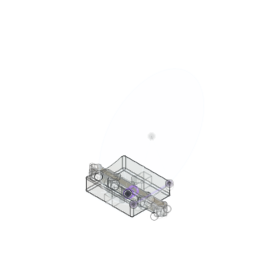
AdjustableDumbbellStand (Autodesk Fusion 360 design; units mm, degrees)
Autodesk Fusion 360 part; units mm, degrees
sketch "Sketch1" plane through (0, 0, 0) normal (0, 0, 1) x (1, 0, 0) in component "Connector"
  line L0 (124.9, -14.9) -> (-124.9, -14.9)
  line L1 (-124.9, -14.9) -> (-124.9, 14.9)
  line L2 (-124.9, 14.9) -> (124.9, 14.9)
  line L3 (124.9, 14.9) -> (124.9, -14.9)
  line L4 (124.9, -14.9) -> (-124.9, 14.9) construction
  line L5 (-124.9, -14.9) -> (124.9, 14.9) construction
  line L6 (124.9, 24.9) -> (124.9, -24.9)
  line L7 (0, 0) -> (144.7, 0) construction
  line L8 (124.9, 24.9) -> (144.7, 0)
  line L9 (124.9, -24.9) -> (144.7, 0)
  line L10 (0, 2.5) -> (0, 20)
  line L11 (-124.9, 24.9) -> (-144.7, 0)
  line L12 (-124.9, -24.9) -> (-144.7, 0)
  line L13 (-124.9, 24.9) -> (-124.9, -24.9)
  line L14 (-124.9, -24.9) -> (-105.1, 0)
  line L15 (-124.9, 24.9) -> (-105.1, 0)
  line L16 (124.9, 24.9) -> (105.1, 0)
  line L17 (124.9, -24.9) -> (105.1, 0)
  dimension "d1" = 249.8
  dimension "d2" = 29.8
  dimension "d3" = 49.8
  dimension "d24" = 19.8
  constraint horizontal L0
  constraint perpendicular L0 L1
  constraint parallel L0 L2
  constraint parallel L1 L3
  constraint coincident L4 L7.start
  constraint coincident L5 L7.start
  constraint coincident L7.start origin
  constraint parallel L3 L6
  constraint collinear L3 L6
  constraint equal L8 L9
  constraint horizontal L7
  constraint symmetric L6.start L10 L11.start
  constraint symmetric L6.end L10 L12.start
  constraint symmetric L7.end L10 L11.end
  constraint symmetric L11.start L13 L15.start
  constraint symmetric L11.end L13 L14.end
  constraint symmetric L12.start L13 L14.start
  constraint symmetric L3 L6.start L8.start
  constraint symmetric L3 L6.end L9.start
  constraint symmetric L3 L7.end L16.end
  constraint collinear L1 L13
  measures "d1" distance of L1.end L2.end
  measures "d2" distance of L0.end L1.end
  measures "d3" distance of L6.start L6.end
  measures "d24" distance of L6 L7.end
extrude "Extrude1" add sketch "Sketch1" along normal blind 28.8 makes body 1 in component "Connector"
fillet "Fillet1" radius 6 10 edges at (-144.7, 0, 14.4) (144.7, 0, 14.4) (116.9482, 14.9, 14.4) (124.9, 24.9, 14.4) (-116.9482, 14.9, 14.4) (-124.9, 24.9, 14.4) (124.9, -24.9, 14.4) (116.9482, -14.9, 14.4) (-124.9, -24.9, 14.4) (-116.9482, -14.9, 14.4) on bodies 1 in component "Connector"
chamfer "Chamfer1" distance 5 angle 45 1 faces at (-38.0179, -4.9667, 28.8) on bodies 1 in component "Connector"
sketch "Sketch1 (2)" plane through (0, 0, 0) normal (0, 0, 1) x (1, 0, 0) in component "Base"
  line L0 (-90, 75) -> (90, 75)
  line L1 (90, 75) -> (90, -75)
  line L2 (90, -75) -> (-90, -75)
  line L3 (-90, -75) -> (-90, 75)
  line L4 (-90, 75) -> (90, -75) construction
  line L5 (90, 75) -> (-90, -75) construction
  line L6 (0, 0) -> (-90, 0) construction
  line L7 (0, 0) -> (0, -75) construction
  dimension "d10" = 180
  dimension "d11" = 150
  constraint horizontal L0
  constraint perpendicular L0 L1
  constraint parallel L0 L2
  constraint parallel L1 L3
  constraint coincident L4 L6.start
  constraint coincident L5 L6.start
  constraint coincident L6.start L7.start
  constraint midpoint L3 L6.end
  constraint midpoint L2 L7.end
  measures "d10" distance of L1.end L2.end
  measures "d11" distance of L0.end L1.end
extrude "Extrude1'" add sketch "Sketch1 (2)" along normal blind 50 separate body makes body 2 in component "Base"
fillet "Fillet1'" radius 6 4 edges at (90, 75, 25) (-90, 75, 25) (-90, -75, 25) (90, -75, 25) on bodies 2 in component "Base"
chamfer "Chamfer1'" distance 5 angle 45 2 faces at (28, -25, 0) (28, -25, 50) on bodies 2 in component "Base"
sketch "Sketch2" plane through (90, 0, 0) normal (1, 0, 0) x (0, 1, 0) in component "Base"
  line L0 (69, 45) -> (-69, 45)
  line L1 (-69, 45) -> (-69, 5)
  line L2 (-69, 5) -> (69, 5)
  line L3 (69, 5) -> (69, 45)
  line L4 (-69, 45) -> (69, 45)
  line L5 (-69, 45) -> (0, 235) construction
  line L6 (0, 235) -> (69, 45) construction
  circle A0 centre (0, 235) radius 200
  line L7 (-69, 35) -> (69, 35) construction
  line L8 (-69, 45) -> (-69, 35) construction
  dimension "d17" = 400
  dimension "d18" = 10
  constraint coincident L0.end L1.start
  constraint coincident L0.start L3.end
  constraint equal L5 L6
  constraint coincident L5.end L6.start
  constraint perpendicular L1 L7
  constraint equal L0 L7
  constraint perpendicular L0 L8
  constraint tangent A0 L7
  measures "d17" diameter of A0
  measures "d18" distance of L0.end L7.start
extrude "Extrude2" cut sketch "Sketch2" against normal through all contours L0 L4 A0 | L0 L4 A0 bodies 2 in component "Base"
sketch "Sketch1 (3)" plane through (0, 0, 0) normal (0, 0, 1) x (1, 0, 0) in component "ConnectorTip"
  line L0 (0, 0) -> (0, -24.9) construction
  line L1 (0, 0) -> (0, 24.9) construction
  line L2 (0, 0) -> (19.8, 0) construction
  line L3 (0, 0) -> (-19.8, 0) construction
  line L4 (0, -24.9) -> (19.8, 0)
  line L5 (0, 24.9) -> (19.8, 0)
  line L6 (0, 24.9) -> (-19.8, 0)
  line L7 (0, -24.9) -> (-19.8, 0)
  line L8 (-7.9518, -14.9) -> (-37.7518, -14.9)
  line L9 (-37.7518, -14.9) -> (-37.7518, 14.9)
  line L10 (-37.7518, 14.9) -> (-7.9518, 14.9)
  line L11 (-7.9518, 14.9) -> (-7.9518, -14.9)
  dimension "d33" = 24.9
  dimension "d34" = 19.8
  dimension "d39" = 29.8
  constraint coincident L0.start L1.start
  constraint vertical L0
  constraint parallel L0 L1
  constraint equal L0 L1
  constraint perpendicular L1 L2
  constraint perpendicular L1 L3
  constraint equal L2 L3
  constraint horizontal L8
  constraint vertical L9
  constraint horizontal L10
  constraint vertical L11
  constraint coincident L7 L8.start
  constraint coincident L6 L10.end
  constraint equal L8 L11
  measures "d33" distance of L0.start L0.end
  measures "d34" distance of L0.start L2.end
  measures "d39" distance of L8.start L10.end
extrude "Extrude1''" add sketch "Sketch1 (3)" along normal blind 28.8 separate body makes body 3 in component "ConnectorTip"
fillet "Fillet1''" radius 6 3 edges at (0, 24.9, 14.4) (19.8, 0, 14.4) (0, -24.9, 14.4) on bodies 3 in component "ConnectorTip"
sketch "Sketch1 (4)" plane through (0, 0, 0) normal (0, 0, 1) x (1, 0, 0) in component "Base (1)"
  line L0 (-90, 75) -> (90, 75)
  line L1 (90, 75) -> (90, -75)
  line L2 (90, -75) -> (-90, -75)
  line L3 (-90, -75) -> (-90, 75)
  line L4 (-90, 75) -> (90, -75) construction
  line L5 (90, 75) -> (-90, -75) construction
  line L6 (0, 0) -> (-90, 0) construction
  line L7 (0, 0) -> (0, -75) construction
  dimension "d10_1" = 180
  dimension "d11_1" = 150
  constraint horizontal L0
  constraint perpendicular L0 L1
  constraint parallel L0 L2
  constraint parallel L1 L3
  constraint coincident L4 L6.start
  constraint coincident L5 L6.start
  constraint coincident L6.start L7.start
  constraint midpoint L3 L6.end
  constraint midpoint L2 L7.end
  measures "d10_1" distance of L1.end L2.end
  measures "d11_1" distance of L0.end L1.end
extrude "Extrude1'''" add sketch "Sketch1 (4)" along normal blind 50 separate body makes body 4 in component "Base (1)"
fillet "Fillet1'''" radius 6 4 edges at (90, 75, 25) (-90, 75, 25) (-90, -75, 25) (90, -75, 25) on bodies 4 in component "Base (1)"
chamfer "Chamfer1''" distance 5 angle 45 2 faces at (28, -25, 0) (28, -25, 50) on bodies 4 in component "Base (1)"
sketch "Sketch2 (2)" plane through (90, 0, 0) normal (1, 0, 0) x (0, 1, 0) in component "Base (1)"
  line L0 (69, 45) -> (-69, 45)
  line L1 (-69, 45) -> (-69, 5)
  line L2 (-69, 5) -> (69, 5)
  line L3 (69, 5) -> (69, 45)
  line L4 (-69, 45) -> (69, 45)
  line L5 (-69, 45) -> (0, 235) construction
  line L6 (0, 235) -> (69, 45) construction
  circle A0 centre (0, 235) radius 200
  line L7 (-69, 35) -> (69, 35) construction
  line L8 (-69, 45) -> (-69, 35) construction
  dimension "d17_1" = 400
  dimension "d18_1" = 10
  constraint coincident L0.end L1.start
  constraint coincident L0.start L3.end
  constraint equal L5 L6
  constraint coincident L5.end L6.start
  constraint perpendicular L1 L7
  constraint equal L0 L7
  constraint perpendicular L0 L8
  constraint tangent A0 L7
  measures "d17_1" diameter of A0
  measures "d18_1" distance of L0.end L7.start
extrude "Extrude2'" cut sketch "Sketch2 (2)" against normal through all contours L0 L4 A0 | L0 L4 A0 bodies 4 in component "Base (1)"
sketch "Sketch1 (5)" plane through (0, 0, 0) normal (0, 0, 1) x (1, 0, 0) in component "ConnectorTip (1)"
  line L0 (0, 0) -> (0, -24.9) construction
  line L1 (0, 0) -> (0, 24.9) construction
  line L2 (0, 0) -> (19.8, 0) construction
  line L3 (0, 0) -> (-19.8, 0) construction
  line L4 (0, -24.9) -> (19.8, 0)
  line L5 (0, 24.9) -> (19.8, 0)
  line L6 (0, 24.9) -> (-19.8, 0)
  line L7 (0, -24.9) -> (-19.8, 0)
  line L8 (-7.9518, -14.9) -> (-37.7518, -14.9)
  line L9 (-37.7518, -14.9) -> (-37.7518, 14.9)
  line L10 (-37.7518, 14.9) -> (-7.9518, 14.9)
  line L11 (-7.9518, 14.9) -> (-7.9518, -14.9)
  dimension "d33_1" = 24.9
  dimension "d34_1" = 19.8
  dimension "d39_1" = 29.8
  constraint coincident L0.start L1.start
  constraint vertical L0
  constraint parallel L0 L1
  constraint equal L0 L1
  constraint perpendicular L1 L2
  constraint perpendicular L1 L3
  constraint equal L2 L3
  constraint horizontal L8
  constraint vertical L9
  constraint horizontal L10
  constraint vertical L11
  constraint coincident L7 L8.start
  constraint coincident L6 L10.end
  constraint equal L8 L11
  measures "d33_1" distance of L0.start L0.end
  measures "d34_1" distance of L0.start L2.end
  measures "d39_1" distance of L8.start L10.end
extrude "Extrude1''''" add sketch "Sketch1 (5)" along normal blind 28.8 separate body makes body 5 in component "ConnectorTip (1)"
fillet "Fillet1''''" radius 6 3 edges at (0, 24.9, 14.4) (19.8, 0, 14.4) (0, -24.9, 14.4) on bodies 5 in component "ConnectorTip (1)"
sketch "Sketch1 (6)" plane through (0, 0, 0) normal (0, 0, 1) x (1, 0, 0) in component "ConnectorTip (2)"
  line L0 (0, 0) -> (0, -24.9) construction
  line L1 (0, 0) -> (0, 24.9) construction
  line L2 (0, 0) -> (19.8, 0) construction
  line L3 (0, 0) -> (-19.8, 0) construction
  line L4 (0, -24.9) -> (19.8, 0)
  line L5 (0, 24.9) -> (19.8, 0)
  line L6 (0, 24.9) -> (-19.8, 0)
  line L7 (0, -24.9) -> (-19.8, 0)
  line L8 (-7.9518, -14.9) -> (-37.7518, -14.9)
  line L9 (-37.7518, -14.9) -> (-37.7518, 14.9)
  line L10 (-37.7518, 14.9) -> (-7.9518, 14.9)
  line L11 (-7.9518, 14.9) -> (-7.9518, -14.9)
  dimension "d33_2" = 24.9
  dimension "d34_2" = 19.8
  dimension "d39_2" = 29.8
  constraint coincident L0.start L1.start
  constraint vertical L0
  constraint parallel L0 L1
  constraint equal L0 L1
  constraint perpendicular L1 L2
  constraint perpendicular L1 L3
  constraint equal L2 L3
  constraint horizontal L8
  constraint vertical L9
  constraint horizontal L10
  constraint vertical L11
  constraint coincident L7 L8.start
  constraint coincident L6 L10.end
  constraint equal L8 L11
  measures "d33_2" distance of L0.start L0.end
  measures "d34_2" distance of L0.start L2.end
  measures "d39_2" distance of L8.start L10.end
extrude "Extrude1'''''" add sketch "Sketch1 (6)" along normal blind 28.8 separate body makes body 6 in component "ConnectorTip (2)"
fillet "Fillet1'''''" radius 6 3 edges at (0, 24.9, 14.4) (19.8, 0, 14.4) (0, -24.9, 14.4) on bodies 6 in component "ConnectorTip (2)"
combine "Combine10" operation cut target body 4 tool bodies 6 5 body 6 seen with x (1, 0, 0) y (0, 1, 0) z (0, 0, 1) at (-52.2482, 0, 0) body 5 seen with x (0, -1, 0) y (1, 0, 0) z (0, 0, 1) at (0, 37.2482, 0) in component "Base (1)"
sketch "Sketch1 (7)" plane through (0, 0, 0) normal (0, 0, 1) x (1, 0, 0) in component "Base (2)"
  line L0 (-90, 75) -> (90, 75)
  line L1 (90, 75) -> (90, -75)
  line L2 (90, -75) -> (-90, -75)
  line L3 (-90, -75) -> (-90, 75)
  line L4 (-90, 75) -> (90, -75) construction
  line L5 (90, 75) -> (-90, -75) construction
  line L6 (0, 0) -> (-90, 0) construction
  line L7 (0, 0) -> (0, -75) construction
  dimension "d10_2" = 180
  dimension "d11_2" = 150
  constraint horizontal L0
  constraint perpendicular L0 L1
  constraint parallel L0 L2
  constraint parallel L1 L3
  constraint coincident L4 L6.start
  constraint coincident L5 L6.start
  constraint coincident L6.start L7.start
  constraint midpoint L3 L6.end
  constraint midpoint L2 L7.end
  measures "d10_2" distance of L1.end L2.end
  measures "d11_2" distance of L0.end L1.end
extrude "Extrude1''''''" add sketch "Sketch1 (7)" along normal blind 50 separate body makes body 7 in component "Base (2)"
fillet "Fillet1''''''" radius 6 4 edges at (90, 75, 25) (-90, 75, 25) (-90, -75, 25) (90, -75, 25) on bodies 7 in component "Base (2)"
chamfer "Chamfer1'''" distance 5 angle 45 2 faces at (28, -25, 0) (28, -25, 50) on bodies 7 in component "Base (2)"
sketch "Sketch2 (3)" plane through (90, 0, 0) normal (1, 0, 0) x (0, 1, 0) in component "Base (2)"
  line L0 (69, 45) -> (-69, 45)
  line L1 (-69, 45) -> (-69, 5)
  line L2 (-69, 5) -> (69, 5)
  line L3 (69, 5) -> (69, 45)
  line L4 (-69, 45) -> (69, 45)
  line L5 (-69, 45) -> (0, 235) construction
  line L6 (0, 235) -> (69, 45) construction
  circle A0 centre (0, 235) radius 200
  line L7 (-69, 35) -> (69, 35) construction
  line L8 (-69, 45) -> (-69, 35) construction
  dimension "d17_2" = 400
  dimension "d18_2" = 10
  constraint coincident L0.end L1.start
  constraint coincident L0.start L3.end
  constraint equal L5 L6
  constraint coincident L5.end L6.start
  constraint perpendicular L1 L7
  constraint equal L0 L7
  constraint perpendicular L0 L8
  constraint tangent A0 L7
  measures "d17_2" diameter of A0
  measures "d18_2" distance of L0.end L7.start
extrude "Extrude2''" cut sketch "Sketch2 (3)" against normal through all contours L0 L4 A0 | L0 L4 A0 bodies 7 in component "Base (2)"
sketch "Sketch1 (8)" plane through (0, 0, 0) normal (0, 0, 1) x (1, 0, 0) in component "ConnectorTip (3)"
  line L0 (0, 0) -> (0, -24.9) construction
  line L1 (0, 0) -> (0, 24.9) construction
  line L2 (0, 0) -> (19.8, 0) construction
  line L3 (0, 0) -> (-19.8, 0) construction
  line L4 (0, -24.9) -> (19.8, 0)
  line L5 (0, 24.9) -> (19.8, 0)
  line L6 (0, 24.9) -> (-19.8, 0)
  line L7 (0, -24.9) -> (-19.8, 0)
  line L8 (-7.9518, -14.9) -> (-37.7518, -14.9)
  line L9 (-37.7518, -14.9) -> (-37.7518, 14.9)
  line L10 (-37.7518, 14.9) -> (-7.9518, 14.9)
  line L11 (-7.9518, 14.9) -> (-7.9518, -14.9)
  dimension "d33_3" = 24.9
  dimension "d34_3" = 19.8
  dimension "d39_3" = 29.8
  constraint coincident L0.start L1.start
  constraint vertical L0
  constraint parallel L0 L1
  constraint equal L0 L1
  constraint perpendicular L1 L2
  constraint perpendicular L1 L3
  constraint equal L2 L3
  constraint horizontal L8
  constraint vertical L9
  constraint horizontal L10
  constraint vertical L11
  constraint coincident L7 L8.start
  constraint coincident L6 L10.end
  constraint equal L8 L11
  measures "d33_3" distance of L0.start L0.end
  measures "d34_3" distance of L0.start L2.end
  measures "d39_3" distance of L8.start L10.end
extrude "Extrude1'''''''" add sketch "Sketch1 (8)" along normal blind 28.8 separate body makes body 8 in component "ConnectorTip (3)"
fillet "Fillet1'''''''" radius 6 3 edges at (0, 24.9, 14.4) (19.8, 0, 14.4) (0, -24.9, 14.4) on bodies 8 in component "ConnectorTip (3)"
sketch "Sketch1 (9)" plane through (0, 0, 0) normal (0, 0, 1) x (1, 0, 0) in component "ConnectorTip (4)"
  line L0 (0, 0) -> (0, -24.9) construction
  line L1 (0, 0) -> (0, 24.9) construction
  line L2 (0, 0) -> (19.8, 0) construction
  line L3 (0, 0) -> (-19.8, 0) construction
  line L4 (0, -24.9) -> (19.8, 0)
  line L5 (0, 24.9) -> (19.8, 0)
  line L6 (0, 24.9) -> (-19.8, 0)
  line L7 (0, -24.9) -> (-19.8, 0)
  line L8 (-7.9518, -14.9) -> (-37.7518, -14.9)
  line L9 (-37.7518, -14.9) -> (-37.7518, 14.9)
  line L10 (-37.7518, 14.9) -> (-7.9518, 14.9)
  line L11 (-7.9518, 14.9) -> (-7.9518, -14.9)
  dimension "d33_4" = 24.9
  dimension "d34_4" = 19.8
  dimension "d39_4" = 29.8
  constraint coincident L0.start L1.start
  constraint vertical L0
  constraint parallel L0 L1
  constraint equal L0 L1
  constraint perpendicular L1 L2
  constraint perpendicular L1 L3
  constraint equal L2 L3
  constraint horizontal L8
  constraint vertical L9
  constraint horizontal L10
  constraint vertical L11
  constraint coincident L7 L8.start
  constraint coincident L6 L10.end
  constraint equal L8 L11
  measures "d33_4" distance of L0.start L0.end
  measures "d34_4" distance of L0.start L2.end
  measures "d39_4" distance of L8.start L10.end
extrude "Extrude1''''''''" add sketch "Sketch1 (9)" along normal blind 28.8 separate body makes body 9 in component "ConnectorTip (4)"
fillet "Fillet1''''''''" radius 6 3 edges at (0, 24.9, 14.4) (19.8, 0, 14.4) (0, -24.9, 14.4) on bodies 9 in component "ConnectorTip (4)"
combine "Combine10'" operation cut target body 7 tool bodies 9 8 body 9 seen with x (1, 0, 0) y (0, 1, 0) z (0, 0, 1) at (-52.2482, 0, 0) body 8 seen with x (0, 1, 0) y (-1, 0, 0) z (0, 0, 1) at (0, -37.2482, 0) in component "Base (2)"
sketch "Sketch1 (10)" plane through (0, 0, 0) normal (0, 0, 1) x (1, 0, 0) in component "Connector_Extender_A_Full_Length"
  line L0 (124.9, -14.9) -> (-124.9, -14.9)
  line L1 (-124.9, -14.9) -> (-124.9, 14.9) construction
  line L2 (-124.9, 14.9) -> (124.9, 14.9)
  line L3 (124.9, 14.9) -> (124.9, -14.9)
  line L4 (124.9, -14.9) -> (-124.9, 14.9) construction
  line L5 (-124.9, -14.9) -> (124.9, 14.9) construction
  line L6 (124.9, 24.9) -> (124.9, -24.9)
  line L7 (0, 0) -> (144.7, 0) construction
  line L8 (124.9, 24.9) -> (144.7, 0)
  line L9 (124.9, -24.9) -> (144.7, 0)
  line L10 (0, 2.5) -> (0, 20)
  line L11 (124.9, -24.9) -> (105.1, 0)
  line L12 (124.9, 24.9) -> (105.1, 0)
  circle A0 centre (-119.9333, -9.9333) radius 4.9667
  circle A1 centre (-119.9333, 9.9333) radius 4.9667
  circle A2 centre (-112.4833, 0) radius 7.45 construction
  arc A3 (-116.9534, -5.96) -> (-116.9534, 5.96) centre (-112.4835, 0) ccw
  line L13 (-124.9, -14.9) -> (-124.9, -9.9333)
  line L14 (-124.9, 9.9333) -> (-124.9, 14.9)
  circle A4 centre (-129.8667, -9.9333) radius 4.9667
  circle A5 centre (-129.8667, 9.9333) radius 4.9667
  circle A6 centre (-137.3167, 0) radius 7.45
  dimension "d1_1" = 249.8
  dimension "d2_1" = 29.8
  dimension "d3_1" = 49.8
  dimension "d24_1" = 19.8
  dimension "d56" = 9.9333
  dimension "d57" = 14.9
  constraint horizontal L0
  constraint perpendicular L0 L1
  constraint parallel L0 L2
  constraint parallel L1 L3
  constraint coincident L4 L7.start
  constraint coincident L5 L7.start
  constraint coincident L7.start origin
  constraint parallel L3 L6
  constraint equal L8 L9
  constraint horizontal L7
  constraint symmetric L3 L6.start L8.start
  constraint symmetric L3 L6.end L9.start
  constraint symmetric L3 L7.end L11.end
  constraint tangent L0 A0
  constraint tangent L1 A0
  constraint symmetric L7 A0 A1
  constraint tangent A0 A2
  constraint tangent A1 A2
  constraint tangent A1 A3
  constraint coincident A1 A3.end
  constraint coincident A2 A3.end
  constraint coincident A0 A3.start
  constraint coincident A2 A3.start
  constraint coincident L1 L13.end
  constraint coincident A0 L13.end
  constraint coincident A1 L14.start
  constraint coincident L1 L14.start
  constraint symmetric L1 A0 A4
  constraint symmetric L1 A1 A5
  constraint symmetric L1 A2 A6
  constraint coincident L6 L9.start
  measures "d1_1" distance of L1.end L2.end
  measures "d2_1" distance of L0.end L1.end
  measures "d3_1" distance of L6.start L6.end
  measures "d24_1" distance of L6 L7.end
  measures "d56" diameter of A0
  measures "d57" diameter of A2
extrude "Extrude1'''''''''" add sketch "Sketch1 (10)" along normal blind 28.8 separate body contours L0 L6 L11 | L0 L2 L3 L6 L11 L12 | L3 L6 L8 L9 | L0 L2 L11 L12 A0 A1 A3 | L2 L6 L12 | L0 A0 L13 | A0 | A0 A1 A3 A4 A5 A6 | A6 | L2 A1 L14 | A1 makes body 10 in component "Connector_Extender_A_Full_Length"
fillet "Fillet1'''''''''" radius 6 5 edges at (144.7, 0, 14.4) (124.9, 24.9, 14.4) (116.9482, 14.9, 14.4) (124.9, -24.9, 14.4) (116.9482, -14.9, 14.4) on bodies 10 in component "Connector_Extender_A_Full_Length"
chamfer "Chamfer1''''" distance 5 angle 45 7 edges at (-3.9759, 14.9, 28.8) (-3.9759, -14.9, 28.8) (135.6634, -11.3642, 28.8) (143.0343, 0, 28.8) (135.6634, 11.3642, 28.8) (119.4768, -18.0799, 28.8) (119.4768, 18.0799, 28.8) on bodies 10 in component "Connector_Extender_A_Full_Length"
sketch "Sketch1 (11)" plane through (0, 0, 0) normal (0, 0, 1) x (1, 0, 0) in component "Connector_Extender_C_Full_Length"
  line L0 (124.9, -14.9) -> (-124.9, -14.9)
  line L1 (-124.9, -14.9) -> (-124.9, 14.9) construction
  line L2 (-124.9, 14.9) -> (124.9, 14.9)
  line L3 (124.9, 14.9) -> (124.9, -14.9)
  line L4 (124.9, -14.9) -> (-124.9, 14.9) construction
  line L5 (-124.9, -14.9) -> (124.9, 14.9) construction
  line L6 (0, 0) -> (124.9, 0) construction
  line L7 (0, 2.5) -> (0, 20)
  circle A0 centre (-119.9333, -9.9333) radius 4.9667
  circle A1 centre (-119.9333, 9.9333) radius 4.9667
  circle A2 centre (-112.4833, 0) radius 7.45 construction
  arc A3 (-116.9533, -5.96) -> (-116.9533, 5.96) centre (-112.4833, 0) ccw
  line L8 (-124.9, -14.9) -> (-124.9, -9.9333)
  line L9 (-124.9, 9.9333) -> (-124.9, 14.9)
  arc A4 (116.9533, 5.96) -> (116.9533, -5.96) centre (112.4833, 0) ccw construction
  circle A5 centre (119.9333, -9.9333) radius 4.9667 construction
  circle A6 centre (119.9333, 9.9333) radius 4.9667 construction
  circle A7 centre (129.8667, -9.9333) radius 4.9667 construction
  circle A8 centre (129.8667, 9.9333) radius 4.9667 construction
  arc A9 (132.8467, -5.96) -> (132.8467, 5.96) centre (137.3167, 0) ccw
  arc A10 (132.8467, -5.96) -> (124.9, -9.9333) centre (129.8667, -9.9333) ccw
  arc A11 (124.9, 9.9333) -> (132.8467, 5.96) centre (129.8667, 9.9333) ccw
  point P0 (-124.9, 0)
  dimension "d1_1_1" = 249.8
  dimension "d2_1_1" = 29.8
  dimension "d56_1" = 9.9333
  dimension "d57_1" = 14.9
  constraint horizontal L0
  constraint perpendicular L0 L1
  constraint parallel L0 L2
  constraint parallel L1 L3
  constraint coincident L4 L6.start
  constraint coincident L5 L6.start
  constraint coincident L6.start origin
  constraint horizontal L6
  constraint tangent L0 A0
  constraint tangent L1 A0
  constraint symmetric L6 A0 A1
  constraint tangent A0 A2
  constraint tangent A1 A2
  constraint tangent A1 A3
  constraint coincident A1 A3.end
  constraint coincident A2 A3.end
  constraint coincident A0 A3.start
  constraint coincident A2 A3.start
  constraint coincident L1 L8.end
  constraint coincident A0 L8.end
  constraint coincident A1 L9.start
  constraint coincident L1 L9.start
  constraint midpoint L3 L6.end
  constraint symmetric L6.end L7 P0
  constraint symmetric L7 A0 A5
  constraint symmetric L7 A1 A6
  constraint symmetric L7 A3.start A4.end
  constraint symmetric L7 A3.end A4.start
  constraint symmetric L7 A3 A4
  constraint symmetric L3 A4.end A9.start
  constraint symmetric L3 A4.start A9.end
  constraint symmetric L3 A4 A9
  constraint symmetric L3 A5 A7
  constraint symmetric L3 A6 A8
  constraint tangent A5 A10
  constraint tangent L3 A10
  constraint coincident L3 A10.end
  constraint tangent A6 A11
  constraint tangent L3 A11
  constraint coincident L3 A11.start
  measures "d1_1_1" distance of L1.end L2.end
  measures "d2_1_1" distance of L0.end L1.end
  measures "d56_1" diameter of A0
  measures "d57_1" diameter of A2
extrude "Extrude1''''''''''" add sketch "Sketch1 (11)" along normal blind 28.8 separate body makes body 11 in component "Connector_Extender_C_Full_Length"
chamfer "Chamfer1'''''" distance 5 angle 45 2 edges at (0, 14.9, 28.8) (0, -14.9, 28.8) on bodies 11 in component "Connector_Extender_C_Full_Length"
sketch "Sketch1 (12)" plane through (0, 0, 0) normal (0, 0, 1) x (1, 0, 0) in component "Connector_Extender_B_Full_Length"
  line L0 (124.9, -14.9) -> (-124.9, -14.9)
  line L1 (-124.9, -14.9) -> (-124.9, 14.9) construction
  line L2 (-124.9, 14.9) -> (124.9, 14.9)
  line L3 (124.9, 14.9) -> (124.9, -14.9)
  line L4 (124.9, -14.9) -> (-124.9, 14.9) construction
  line L5 (-124.9, -14.9) -> (124.9, 14.9) construction
  line L6 (124.9, 24.9) -> (124.9, -24.9)
  line L7 (0, 0) -> (144.7, 0) construction
  line L8 (124.9, 24.9) -> (144.7, 0)
  line L9 (124.9, -24.9) -> (144.7, 0)
  line L10 (0, 2.5) -> (0, 20)
  line L11 (124.9, -24.9) -> (105.1, 0)
  line L12 (124.9, 24.9) -> (105.1, 0)
  circle A0 centre (-119.9333, -9.9333) radius 4.9667
  circle A1 centre (-119.9333, 9.9333) radius 4.9667
  circle A2 centre (-112.4833, 0) radius 7.45 construction
  arc A3 (-116.9533, -5.96) -> (-116.9534, 5.9599) centre (-112.4836, 0) ccw
  line L13 (-124.9, -14.9) -> (-124.9, -9.9333)
  line L14 (-124.9, 9.9333) -> (-124.9, 14.9)
  dimension "d1_1_2_1" = 249.8
  dimension "d2_1_2_1" = 29.8
  dimension "d3_1_2_1" = 49.8
  dimension "d24_1_2_1" = 19.8
  dimension "d56_2_1" = 9.9333
  dimension "d57_2_1" = 14.9
  constraint horizontal L0
  constraint perpendicular L0 L1
  constraint parallel L0 L2
  constraint parallel L1 L3
  constraint coincident L4 L7.start
  constraint coincident L5 L7.start
  constraint coincident L7.start origin
  constraint parallel L3 L6
  constraint equal L8 L9
  constraint horizontal L7
  constraint symmetric L3 L6.start L8.start
  constraint symmetric L3 L6.end L9.start
  constraint symmetric L3 L7.end L11.end
  constraint tangent L0 A0
  constraint tangent L1 A0
  constraint symmetric L7 A0 A1
  constraint tangent A0 A2
  constraint tangent A1 A2
  constraint tangent A1 A3
  constraint coincident A1 A3.end
  constraint coincident A2 A3.end
  constraint coincident A0 A3.start
  constraint coincident A2 A3.start
  constraint coincident L1 L13.end
  constraint coincident A0 L13.end
  constraint coincident A1 L14.start
  constraint coincident L1 L14.start
  constraint coincident L0.start L6
  measures "d1_1_2_1" distance of L1.end L2.end
  measures "d2_1_2_1" distance of L0.end L1.end
  measures "d3_1_2_1" distance of L6.start L6.end
  measures "d24_1_2_1" distance of L6 L7.end
  measures "d56_2_1" diameter of A0
  measures "d57_2_1" diameter of A2
extrude "Extrude1'''''''''''" add sketch "Sketch1 (12)" along normal blind 28.8 separate body makes body 12 in component "Connector_Extender_B_Full_Length"
fillet "Fillet1''''''''''" radius 6 5 edges at (144.7, 0, 14.4) (124.9, 24.9, 14.4) (116.9482, 14.9, 14.4) (116.9482, -14.9, 14.4) (124.9, -24.9, 14.4) on bodies 12 in component "Connector_Extender_B_Full_Length"
chamfer "Chamfer1''''''" distance 5 angle 45 11 edges at (-5.4232, 14.9, 28.8) (116.6607, 15.496, 28.8) (119.4768, 18.0799, 28.8) (124.9, 21.2598, 28.8) (135.6634, 11.3642, 28.8) (143.0343, 0, 28.8) (135.6634, -11.3642, 28.8) (124.9, -21.2598, 28.8) (119.4768, -18.0799, 28.8) (116.6607, -15.496, 28.8) (-5.4232, -14.9, 28.8) on bodies 12 in component "Connector_Extender_B_Full_Length"
sketch "Sketch1 (13)" plane through (0, 0, 0) normal (0, 0, 1) x (1, 0, 0) in component "Connector_Extender_C_Half_Length"
  line L0 (62.45, -14.9) -> (-62.45, -14.9)
  line L1 (-62.45, -14.9) -> (-62.45, 14.9) construction
  line L2 (-62.45, 14.9) -> (62.45, 14.9)
  line L3 (62.45, 14.9) -> (62.45, -14.9)
  line L4 (62.45, -14.9) -> (-62.45, 14.9) construction
  line L5 (-62.45, -14.9) -> (62.45, 14.9) construction
  line L6 (0, 0) -> (62.45, 0) construction
  line L7 (0, 2.5) -> (0, 20)
  circle A0 centre (-57.4833, -9.9333) radius 4.9667
  circle A1 centre (-57.4833, 9.9333) radius 4.9667
  circle A2 centre (-50.0333, 0) radius 7.45 construction
  arc A3 (-54.5033, -5.96) -> (-54.5033, 5.96) centre (-50.0333, 0) ccw
  line L8 (-62.45, -14.9) -> (-62.45, -9.9333)
  line L9 (-62.45, 9.9333) -> (-62.45, 14.9)
  arc A4 (54.5033, 5.96) -> (54.5033, -5.96) centre (50.0333, 0) ccw construction
  circle A5 centre (57.4833, -9.9333) radius 4.9667 construction
  circle A6 centre (57.4833, 9.9333) radius 4.9667 construction
  circle A7 centre (67.4167, -9.9333) radius 4.9667 construction
  circle A8 centre (67.4167, 9.9333) radius 4.9667 construction
  arc A9 (70.3967, -5.96) -> (70.3967, 5.96) centre (74.8667, 0) ccw
  arc A10 (70.3967, -5.96) -> (62.45, -9.9334) centre (67.4167, -9.9334) ccw
  arc A11 (62.45, 9.9334) -> (70.3967, 5.96) centre (67.4167, 9.9334) ccw
  point P0 (-62.45, 0)
  dimension "d1_1_1_1" = 124.9
  dimension "d2_1_1_1" = 29.8
  dimension "d56_1_1" = 9.9333
  dimension "d57_1_1" = 14.9
  constraint horizontal L0
  constraint perpendicular L0 L1
  constraint parallel L0 L2
  constraint parallel L1 L3
  constraint coincident L4 L6.start
  constraint coincident L5 L6.start
  constraint coincident L6.start origin
  constraint horizontal L6
  constraint tangent L0 A0
  constraint tangent L1 A0
  constraint symmetric L6 A0 A1
  constraint tangent A0 A2
  constraint tangent A1 A2
  constraint tangent A1 A3
  constraint coincident A1 A3.end
  constraint coincident A2 A3.end
  constraint coincident A0 A3.start
  constraint coincident A2 A3.start
  constraint coincident L1 L8.end
  constraint coincident A0 L8.end
  constraint coincident A1 L9.start
  constraint coincident L1 L9.start
  constraint midpoint L3 L6.end
  constraint symmetric L6.end L7 P0
  constraint symmetric L7 A0 A5
  constraint symmetric L7 A1 A6
  constraint symmetric L7 A3.start A4.end
  constraint symmetric L7 A3.end A4.start
  constraint symmetric L7 A3 A4
  constraint symmetric L3 A4.end A9.start
  constraint symmetric L3 A4.start A9.end
  constraint symmetric L3 A4 A9
  constraint symmetric L3 A5 A7
  constraint symmetric L3 A6 A8
  constraint tangent A5 A10
  constraint tangent L3 A10
  constraint coincident L3 A10.end
  constraint tangent A6 A11
  constraint tangent L3 A11
  constraint coincident L3 A11.start
  measures "d1_1_1_1" distance of L1.end L2.end
  measures "d2_1_1_1" distance of L0.end L1.end
  measures "d56_1_1" diameter of A0
  measures "d57_1_1" diameter of A2
extrude "Extrude1''''''''''''" add sketch "Sketch1 (13)" along normal blind 28.8 separate body makes body 13 in component "Connector_Extender_C_Half_Length"
chamfer "Chamfer1'''''''" distance 5 angle 45 2 edges at (0, 14.9, 28.8) (0, -14.9, 28.8) on bodies 13 in component "Connector_Extender_C_Half_Length"
sketch "Sketch1 (14)" plane through (0, 0, 0) normal (0, 0, 1) x (1, 0, 0) in component "Connector_Extender_A_Half_Length"
  line L0 (62.45, -14.9) -> (-62.45, -14.9)
  line L1 (-62.45, -14.9) -> (-62.45, 14.9) construction
  line L2 (-62.45, 14.9) -> (62.45, 14.9)
  line L3 (62.45, 14.9) -> (62.45, -14.9)
  line L4 (62.45, -14.9) -> (-62.45, 14.9) construction
  line L5 (-62.45, -14.9) -> (62.45, 14.9) construction
  line L6 (62.45, 24.9) -> (62.45, -24.9)
  line L7 (0, 0) -> (82.25, 0) construction
  line L8 (62.45, 24.9) -> (82.25, 0)
  line L9 (62.45, -24.9) -> (82.25, 0)
  line L10 (0, 2.5) -> (0, 20)
  line L11 (62.45, -24.9) -> (42.65, 0)
  line L12 (62.45, 24.9) -> (42.65, 0)
  circle A0 centre (-57.4833, -9.9333) radius 4.9667
  circle A1 centre (-57.4833, 9.9333) radius 4.9667
  circle A2 centre (-50.0333, 0) radius 7.45 construction
  arc A3 (-54.5033, -5.96) -> (-54.5033, 5.96) centre (-50.0334, 0) ccw
  line L13 (-62.45, -14.9) -> (-62.45, -9.9333)
  line L14 (-62.45, 9.9333) -> (-62.45, 14.9)
  circle A4 centre (-67.4167, -9.9333) radius 4.9667
  circle A5 centre (-67.4167, 9.9333) radius 4.9667
  circle A6 centre (-74.8667, 0) radius 7.45
  dimension "d1_1_2" = 124.9
  dimension "d2_1_2" = 29.8
  dimension "d3_1_1" = 49.8
  dimension "d24_1_1" = 19.8
  dimension "d56_2" = 9.9333
  dimension "d57_2" = 14.9
  constraint horizontal L0
  constraint perpendicular L0 L1
  constraint parallel L0 L2
  constraint parallel L1 L3
  constraint coincident L4 L7.start
  constraint coincident L5 L7.start
  constraint coincident L7.start origin
  constraint parallel L3 L6
  constraint collinear L3 L6
  constraint equal L8 L9
  constraint horizontal L7
  constraint symmetric L3 L6.start L8.start
  constraint symmetric L3 L6.end L9.start
  constraint symmetric L3 L7.end L11.end
  constraint tangent L0 A0
  constraint tangent L1 A0
  constraint symmetric L7 A0 A1
  constraint tangent A0 A2
  constraint tangent A1 A2
  constraint tangent A1 A3
  constraint coincident A1 A3.end
  constraint coincident A2 A3.end
  constraint coincident A0 A3.start
  constraint coincident A2 A3.start
  constraint coincident L1 L13.end
  constraint coincident A0 L13.end
  constraint coincident A1 L14.start
  constraint coincident L1 L14.start
  constraint symmetric L1 A0 A4
  constraint symmetric L1 A1 A5
  constraint symmetric L1 A2 A6
  constraint coincident L6 L9.start
  measures "d1_1_2" distance of L1.end L2.end
  measures "d2_1_2" distance of L0.end L1.end
  measures "d3_1_1" distance of L6.start L6.end
  measures "d24_1_1" distance of L6 L7.end
  measures "d56_2" diameter of A0
  measures "d57_2" diameter of A2
extrude "Extrude1'''''''''''''" add sketch "Sketch1 (14)" along normal blind 28.8 separate body contours L0 L6 L11 | L0 L2 L3 L6 L11 L12 | L3 L6 L8 L9 | L0 L2 L11 L12 A0 A1 A3 | L2 L6 L12 | L0 A0 L13 | A0 | A0 A1 A3 A4 A5 A6 | A6 | L2 A1 L14 | A1 makes body 14 in component "Connector_Extender_A_Half_Length"
fillet "Fillet1'''''''''''" radius 6 5 edges at (82.25, 0, 14.4) (62.45, 24.9, 14.4) (54.4982, 14.9, 14.4) (62.45, -24.9, 14.4) (54.4982, -14.9, 14.4) on bodies 14 in component "Connector_Extender_A_Half_Length"
chamfer "Chamfer1''''''''" distance 5 angle 45 7 edges at (-3.9759, 14.9, 28.8) (-3.9759, -14.9, 28.8) (73.2134, -11.3642, 28.8) (80.5843, 0, 28.8) (73.2134, 11.3642, 28.8) (57.0268, -18.0799, 28.8) (57.0268, 18.0799, 28.8) on bodies 14 in component "Connector_Extender_A_Half_Length"
sketch "Sketch1 (15)" plane through (0, 0, 0) normal (0, 0, 1) x (1, 0, 0) in component "Connector_Extender_B_Half_Length"
  line L0 (62.45, -14.9) -> (-62.45, -14.9)
  line L1 (-62.45, -14.9) -> (-62.45, 14.9) construction
  line L2 (-62.45, 14.9) -> (62.45, 14.9)
  line L3 (62.45, 14.9) -> (62.45, -14.9)
  line L4 (62.45, -14.9) -> (-62.45, 14.9) construction
  line L5 (-62.45, -14.9) -> (62.45, 14.9) construction
  line L6 (62.45, 24.9) -> (62.45, -24.9)
  line L7 (0, 0) -> (82.25, 0) construction
  line L8 (62.45, 24.9) -> (82.25, 0)
  line L9 (62.45, -24.9) -> (82.25, 0)
  line L10 (0, 2.5) -> (0, 20)
  line L11 (62.45, -24.9) -> (42.65, 0)
  line L12 (62.45, 24.9) -> (42.65, 0)
  circle A0 centre (-57.4833, -9.9333) radius 4.9667
  circle A1 centre (-57.4833, 9.9333) radius 4.9667
  circle A2 centre (-50.0333, 0) radius 7.45 construction
  arc A3 (-54.5033, -5.96) -> (-54.5033, 5.96) centre (-50.0334, 0) ccw
  line L13 (-62.45, -14.9) -> (-62.45, -9.9333)
  line L14 (-62.45, 9.9333) -> (-62.45, 14.9)
  dimension "d1_1_2_1_1" = 124.9
  dimension "d2_1_2_1_1" = 29.8
  dimension "d3_1_2_1_1" = 49.8
  dimension "d24_1_2_1_1" = 19.8
  dimension "d56_2_1_1" = 9.9333
  dimension "d57_2_1_1" = 14.9
  constraint horizontal L0
  constraint perpendicular L0 L1
  constraint parallel L0 L2
  constraint parallel L1 L3
  constraint coincident L4 L7.start
  constraint coincident L5 L7.start
  constraint coincident L7.start origin
  constraint parallel L3 L6
  constraint collinear L3 L6
  constraint equal L8 L9
  constraint horizontal L7
  constraint symmetric L3 L6.start L8.start
  constraint symmetric L3 L6.end L9.start
  constraint symmetric L3 L7.end L11.end
  constraint tangent L0 A0
  constraint tangent L1 A0
  constraint symmetric L7 A0 A1
  constraint tangent A0 A2
  constraint tangent A1 A2
  constraint tangent A1 A3
  constraint coincident A1 A3.end
  constraint coincident A2 A3.end
  constraint coincident A0 A3.start
  constraint coincident A2 A3.start
  constraint coincident L1 L13.end
  constraint coincident A0 L13.end
  constraint coincident A1 L14.start
  constraint coincident L1 L14.start
  constraint coincident L0.start L6
  constraint tangent A0 L13
  constraint tangent A0 A3
  measures "d1_1_2_1_1" distance of L1.end L2.end
  measures "d2_1_2_1_1" distance of L0.end L1.end
  measures "d3_1_2_1_1" distance of L6.start L6.end
  measures "d24_1_2_1_1" distance of L6 L7.end
  measures "d56_2_1_1" diameter of A0
  measures "d57_2_1_1" diameter of A2
extrude "Extrude1''''''''''''''" add sketch "Sketch1 (15)" along normal blind 28.8 separate body makes body 15 in component "Connector_Extender_B_Half_Length"
fillet "Fillet1''''''''''''" radius 6 5 edges at (82.25, 0, 14.4) (62.45, 24.9, 14.4) (54.4982, 14.9, 14.4) (54.4982, -14.9, 14.4) (62.45, -24.9, 14.4) on bodies 15 in component "Connector_Extender_B_Half_Length"
chamfer "Chamfer1'''''''''" distance 5 angle 45 11 edges at (-5.4232, 14.9, 28.8) (54.2107, 15.496, 28.8) (57.0268, 18.0799, 28.8) (62.45, 21.2598, 28.8) (73.2134, 11.3642, 28.8) (80.5843, 0, 28.8) (73.2134, -11.3642, 28.8) (62.45, -21.2598, 28.8) (57.0268, -18.0799, 28.8) (54.2107, -15.496, 28.8) (-5.4232, -14.9, 28.8) on bodies 15 in component "Connector_Extender_B_Half_Length"
component "Base" placed x (1, 0, 0) y (0, 1, 0) z (0, 0, 1) at (0, 0, 0)
component "Connector" placed x (1, 0, 0) y (0, 1, 0) z (0, 0, 1) at (0, 0, 0)
component "ConnectorTip" placed x (1, 0, 0) y (0, 1, 0) z (0, 0, 1) at (0, 0, 0)
component "Base_Two_Dumbbells_A" placed x (1, 0, 0) y (0, 1, 0) z (0, 0, 1) at (0, 0, 0)
component "Base_Two_Dumbbells_B" placed x (1, 0, 0) y (0, 1, 0) z (0, 0, 1) at (0, 0, 0)
component "Connector_Extender_A_Full_Length" placed x (1, 0, 0) y (0, 1, 0) z (0, 0, 1) at (0, 0, 0)
component "Connector_Extender_C_Full_Length" placed x (1, 0, 0) y (0, 1, 0) z (0, 0, 1) at (0, 0, 0)
component "Connector_Extender_B_Full_Length" placed x (1, 0, 0) y (0, 1, 0) z (0, 0, 1) at (0, 0, 0)
component "Connector_Extender_C_Half_Length" placed x (1, 0, 0) y (0, 1, 0) z (0, 0, 1) at (0, 0, 0)
component "Connector_Extender_A_Half_Length" placed x (1, 0, 0) y (0, 1, 0) z (0, 0, 1) at (0, 0, 0)
component "Connector_Extender_B_Half_Length" placed x (1, 0, 0) y (0, 1, 0) z (0, 0, 1) at (0, 0, 0)
component "Base (1)" placed x (1, 0, 0) y (0, 1, 0) z (0, 0, 1) at (0, 0, 0) in component "Base_Two_Dumbbells_A"
component "ConnectorTip (1)" placed x (0, -1, 0) y (1, 0, 0) z (0, 0, 1) at (0, 37.2482, 0) in component "Base_Two_Dumbbells_A"
component "ConnectorTip (2)" placed x (1, 0, 0) y (0, 1, 0) z (0, 0, 1) at (-52.2482, 0, 0) in component "Base_Two_Dumbbells_A"
component "Base (2)" placed x (1, 0, 0) y (0, 1, 0) z (0, 0, 1) at (0, 0, 0) in component "Base_Two_Dumbbells_B"
component "ConnectorTip (3)" placed x (0, 1, 0) y (-1, 0, 0) z (0, 0, 1) at (0, -37.2482, 0) in component "Base_Two_Dumbbells_B"
component "ConnectorTip (4)" placed x (1, 0, 0) y (0, 1, 0) z (0, 0, 1) at (-52.2482, 0, 0) in component "Base_Two_Dumbbells_B"
equation "d1 = ConnectorCoreLenght"
equation "d2 = ConnectorWidth"
equation "d3 = ConnectorTipWidth"
equation "d5 = ConnectorHeight"
equation "d8 = ConnectorFilletRadius"
equation "d10 = BaseLength"
equation "d11 = BaseWidth"
equation "d12 = BaseHeight"
equation "d17 = BaseTopCotoutRadius"
equation "d18 = BaseTopCotoutDistance"
equation "ConnectorWidth = 30 mm - Tolerance"
equation "ConnectorHeight = 29 mm - Tolerance"
equation "ConnectorCoreLenght = 250 mm - Tolerance"
equation "ConnectorTipLength = 20 mm - Tolerance"
equation "d24 = ConnectorTipLength"
equation "Tolerance = 0.2 mm"
equation "BaseTopCotoutRadius = 400 mm"
equation "BaseTopCotoutDistance = 10 mm"
equation "BaseWidth = 150 mm"
equation "BaseLength = 180 mm"
equation "BaseHeight = 50 mm"
equation "ConnectorFilletRadius = 6 mm"
equation "ConnectorTipWidth = 50 mm - Tolerance"
equation "d33 = ConnectorTipWidth / 2"
equation "d34 = ConnectorTipLength"
equation "d35 = ConnectorHeight"
equation "d38 = ConnectorFilletRadius"
equation "d39 = ConnectorWidth"
equation "d10_1 = BaseLength"
equation "d11_1 = BaseWidth"
equation "d12_1 = BaseHeight"
equation "d17_1 = BaseTopCotoutRadius"
equation "d18_1 = BaseTopCotoutDistance"
equation "d33_1 = ConnectorTipWidth / 2"
equation "d34_1 = ConnectorTipLength"
equation "d35_1 = ConnectorHeight"
equation "d38_1 = ConnectorFilletRadius"
equation "d39_1 = ConnectorWidth"
equation "d33_2 = ConnectorTipWidth / 2"
equation "d34_2 = ConnectorTipLength"
equation "d35_2 = ConnectorHeight"
equation "d38_2 = ConnectorFilletRadius"
equation "d39_2 = ConnectorWidth"
equation "d10_2 = BaseLength"
equation "d11_2 = BaseWidth"
equation "d12_2 = BaseHeight"
equation "d17_2 = BaseTopCotoutRadius"
equation "d18_2 = BaseTopCotoutDistance"
equation "d33_3 = ConnectorTipWidth / 2"
equation "d34_3 = ConnectorTipLength"
equation "d35_3 = ConnectorHeight"
equation "d38_3 = ConnectorFilletRadius"
equation "d39_3 = ConnectorWidth"
equation "d33_4 = ConnectorTipWidth / 2"
equation "d34_4 = ConnectorTipLength"
equation "d35_4 = ConnectorHeight"
equation "d38_4 = ConnectorFilletRadius"
equation "d39_4 = ConnectorWidth"
equation "d1_1 = ConnectorCoreLenght"
equation "d2_1 = ConnectorWidth"
equation "d3_1 = ConnectorTipWidth"
equation "d5_1 = ConnectorHeight"
equation "d8_1 = ConnectorFilletRadius"
equation "d24_1 = ConnectorTipLength"
equation "d56 = ConnectorWidth / 3"
equation "d57 = ConnectorWidth / 2"
equation "d1_1_1 = ConnectorCoreLenght"
equation "d2_1_1 = ConnectorWidth"
equation "d5_1_1 = ConnectorHeight"
equation "d56_1 = ConnectorWidth / 3"
equation "d57_1 = ConnectorWidth / 2"
equation "d1_1_2_1 = ConnectorCoreLenght"
equation "d2_1_2_1 = ConnectorWidth"
equation "d3_1_2_1 = ConnectorTipWidth"
equation "d5_1_2_1 = ConnectorHeight"
equation "d8_1_2_1 = ConnectorFilletRadius"
equation "d24_1_2_1 = ConnectorTipLength"
equation "d56_2_1 = ConnectorWidth / 3"
equation "d57_2_1 = ConnectorWidth / 2"
equation "d1_1_1_1 = ConnectorCoreLenght / 2"
equation "d2_1_1_1 = ConnectorWidth"
equation "d5_1_1_1 = ConnectorHeight"
equation "d56_1_1 = ConnectorWidth / 3"
equation "d57_1_1 = ConnectorWidth / 2"
equation "d1_1_2 = ConnectorCoreLenght / 2"
equation "d2_1_2 = ConnectorWidth"
equation "d3_1_1 = ConnectorTipWidth"
equation "d5_1_2 = ConnectorHeight"
equation "d8_1_1 = ConnectorFilletRadius"
equation "d24_1_1 = ConnectorTipLength"
equation "d56_2 = ConnectorWidth / 3"
equation "d57_2 = ConnectorWidth / 2"
equation "d1_1_2_1_1 = ConnectorCoreLenght / 2"
equation "d2_1_2_1_1 = ConnectorWidth"
equation "d3_1_2_1_1 = ConnectorTipWidth"
equation "d5_1_2_1_1 = ConnectorHeight"
equation "d8_1_2_1_1 = ConnectorFilletRadius"
equation "d24_1_2_1_1 = ConnectorTipLength"
equation "d56_2_1_1 = ConnectorWidth / 3"
equation "d57_2_1_1 = ConnectorWidth / 2"
